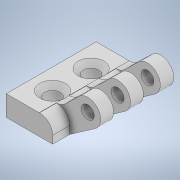
# Autodesk Inventor part: halfhinge
Saved by Autodesk Inventor 2022 (Build 260153000, 153)
## iProperties
Created: 2022-08-02
Part Number: halfhinge
Material: Generic
Document SubType Name: Modeling
Designer: thoma
Density: 1 g/cm^3
Appearance: Default
Author: thoma
Autodesk Inventor part; units mm, degrees
ref_plane "YZ Plane" through (0, 0, 0) normal (1, 0, 0) x (0, 1, 0)
ref_plane "XZ Plane" through (0, 0, 0) normal (0, 1, 0) x (-1, 0, 0)
ref_plane "XY Plane" through (0, 0, 0) normal (0, 0, 1) x (1, 0, 0)
sketch "Sketch2" plane through (0, 0, 0) normal (0, 1, 0) x (-1, 0, 0)
  line L0 (0, 0) -> (20, 0)
  line L1 (20, 0) -> (20, -35)
  line L2 (20, -35) -> (0, -35)
  line L3 (0, -35) -> (0, 0)
  dimension "d0" = 35
  dimension "d1" = 20
  constraints: 8 end point, 2 parallel, 1 horizontal, 1 perpendicular
  measures "d0" distance of L0.end L1.end
  measures "d1" distance of L0.start L0.end
extrude "Extrusion1" add sketch "Sketch2" along normal blind 8
sketch "Sketch3" plane through (0, 0, -35) normal (0, 0, -1) x (-1, 0, 0)
  line L0 (0, 0) -> (20, 0) projected
  line L1 (1.9454, 0) -> (-8.0206, 6.9783)
  line L2 (-8.0206, 6.9783) -> (-2.2848, 15.1698) construction
  line L3 (-2.2848, 15.1698) -> (7.9547, 8)
  line L4 (0, 8) -> (20, 8) projected
  arc A0 (-2.2848, 15.1698) -> (-8.0206, 6.9783) centre (-5.1527, 11.074) ccw
  circle A1 centre (-5.1527, 11.074) radius 2.5
  line L5 (0, 0) -> (0, 8) construction
  line L6 (-5.1527, 11.074) -> (0, 8) construction
  line L7 (1.9454, 0) -> (7.9547, 8)
  line L8 (-2.2848, 15.1698) -> (6.7994, 6.4619)
  dimension "d4" = 5
  dimension "d5" = 10
  dimension "d6" = 6
  dimension "d21" = 35
  constraints: 12 end point, 3 point on line, 2 centre point, 2 point on circle, 1 coincident, 1 midpoint, 1 perpendicular
  measures "d4" diameter of A1
  measures "d5" distance between parallel lines of L1 L3
  measures "d6" distance of L6.start L4.start
  measures "d21" angle of L1 L0
extrude "Extrusion2" add sketch "Sketch3" against normal up to surface (35 mm away) contours L1 A0 L8 L7
sketch "Sketch4" plane through (0, 0, -35) normal (0, 0, -1) x (-1, 0, 0)
  line L0 (-8.0206, 6.9783) -> (0, 1.3622) projected
  line L1 (-4.533, 4.5362) -> (4.5811, -1.8456)
  line L2 (4.5811, -1.8456) -> (-4.9445, -1.8456)
  line L3 (-4.9445, -1.8456) -> (-4.533, 4.5362)
  point P0 (0, 0)
  point P1 (0, 1.3622)
  constraints: 6 end point, 1 collinear, 1 horizontal, 1 point on line
extrude "Extrusion3" cut sketch "Sketch4" against normal up to next
sketch "Sketch5" plane through (0, 8, 0) normal (0, 1, 0) x (1, 0, 0)
  line L0 (-5.1948, 35) -> (-20, 35) construction
  line L1 (-12, 35) -> (-12, 25) construction
  line L2 (-12, 25) -> (-12, 10) construction
  line L3 (-20, 35) -> (-20, 0) construction
  point P0 (0, 0)
  point P1 (-7.9547, 35)
  dimension "d11" = 10
  dimension "d12" = 15
  dimension "d13" = 8
  constraints: 4 end point, 2 coincident, 2 point on line, 1 vertical
  measures "d11" distance of L1.start L1.end
  measures "d12" distance of L1.end L2.end
  measures "d13" distance between parallel lines of L3 L1
hole "Hole1" at (-12, 8, -25) at (-12, 8, -10) direction (0, -1, 0) diameter 6 end through all countersink diameter 10 countersink angle 90
fillet "Fillet1" radius 5 1 edges at (-5.1948, 8, -17.5)
sketch "Sketch6" plane through (0, 0, 0) normal (0, -1, 0) x (1, 0, 0)
  line L0 (8.0206, 0) -> (-1.9454, 0) projected
  line L1 (-1.9454, 0) -> (16.0794, 0)
  line L2 (16.0794, 0) -> (16.0794, -6.6)
  line L3 (16.0794, -6.6) -> (-1.9454, -6.6)
  line L4 (-1.9454, -6.6) -> (-1.9454, 0)
  point P0 (0, 0)
  dimension "d23" = 6.6
  constraints: 8 end point, 2 parallel, 1 horizontal, 1 perpendicular
  measures "d23" distance of L1.end L2.end
extrude "Extrusion4" cut sketch "Sketch6" against normal up to next
fillet "Fillet2" radius 5 1 edges at (-1.9454, 11.1148, -3.3)
pattern_linear "Rectangular Pattern1" count 3 spacing 11.6 along (0, 0, -1) of "Extrusion4", "Fillet2"
body "Solid1"
